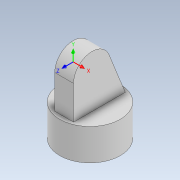
# Autodesk Inventor part: hip_back
Saved by Autodesk Inventor 2020 (Build 240168000, 168)
## iProperties
Created: 2021-01-29
Part Number: hip_back
Material: Generic
Document SubType Name: Modeling
Designer: DELL
Density: 1 g/cm^3
Appearance: Default
Author: DELL
Autodesk Inventor part; units mm, degrees
ref_plane "YZ Plane" through (0, 0, 0) normal (1, 0, 0) x (0, 1, 0)
ref_plane "XZ Plane" through (0, 0, 0) normal (0, 1, 0) x (-1, 0, 0)
ref_plane "XY Plane" through (0, 0, 0) normal (0, 0, 1) x (1, 0, 0)
sketch "Sketch1" plane through (0, 0, 0) normal (1, 0, 0) x (0, 1, 0)
  circle A0 centre (0, 0) radius 27.5
  line L0 (0, 27.5) -> (-50, 27.5)
  line L1 (-50, 27.5) -> (-50, -49.5)
  line L2 (-50, -49.5) -> (10.1699, -25.5504)
  dimension "d0" = 55
  dimension "d1" = 50
  dimension "d2" = 77
  constraints: 6 end point, 2 point on circle, 2 tangent, 1 centre point, 1 coincident, 1 horizontal, 1 perpendicular
  measures "d0" diameter of A0
  measures "d1" distance of L0.start L0.end
  measures "d2" distance of L0.end L1.end
extrude "Extrusion1" add sketch "Sketch1" along normal blind 28
sketch "Sketch2" plane through (0, -50, -49.5) normal (0, -1, 0) x (1, 0, 0)
  circle A0 centre (14, 38.5) radius 45
  line L0 (0, 77) -> (28, 77) projected
  line L1 (0, 77) -> (0, 0) projected
  point P0 (0, 49.5)
  point P1 (14, 77)
  point P2 (0, 38.5)
  dimension "d5" = 90
  constraints: 2 midpoint, 1 centre point, 1 horizontal alignment, 1 vertical alignment
  measures "d5" diameter of A0
extrude "Extrusion2" add sketch "Sketch2" along normal blind 47
sketch "Sketch3" plane through (14, -97, -11) normal (0, -1, 0) x (1, 0, 0)
  circle A0 centre (0, 0) radius 45 projected
  circle A1 centre (0, 0) radius 40
  line L0 (0, 0) -> (-45, 0) construction
  line L1 (0, 0) -> (-38.9711, 22.5) construction
  line L2 (0, 0) -> (-38.9711, -22.5) construction
  line L3 (-34.641, 20) -> (-24.3333, 37.8536)
  line L4 (-34.641, -20) -> (-24.3333, -37.8536)
  point P0 (-14, 11)
  dimension "d14" = 80
  dimension "d15" = 30
  constraints: 10 end point, 7 point on circle, 2 point on line, 2 tangent, 1 centre point, 1 coincident, 1 horizontal, 1 other
  measures "d14" diameter of A1
  measures "d15" angle of L0 L1
body "Solid1"
